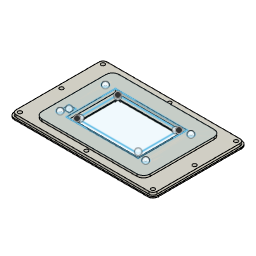
Display Mount - TFT35V20 (Autodesk Fusion 360 design; units mm, degrees)
Autodesk Fusion 360 part; units mm, degrees
note: some values were not read from the file. Set by a fixed rule: which sketch regions a step uses.
sketch "Sketch1" plane through (0, 0, 0) normal (0, 0, 1) x (1, 0, 0)
  circle A0 centre (-81.65, 51) radius 2.3
  circle A1 centre (81.65, 51) radius 2.3
  circle A2 centre (-81.65, -51) radius 2.3
  circle A3 centre (81.65, -51) radius 2.3
  line L0 (-81.65, 51) -> (81.65, 51) construction
  line L1 (81.65, 51) -> (81.65, -51) construction
  line L2 (81.65, -51) -> (-81.65, -51) construction
  line L3 (-81.65, -51) -> (-81.65, 51) construction
  circle A4 centre (-81.65, 0) radius 2.3
  circle A5 centre (0, 51) radius 2.3
  circle A6 centre (81.65, 0) radius 2.3
  circle A7 centre (0, -51) radius 2.3
  line L4 (0, 87.0412) -> (0, 82.962)
  line L5 (0, 82.962) -> (0, -82.962) construction
  line L6 (-123.3001, 0) -> (123.3001, 0) construction
  circle A8 centre (81.65, -51) radius 4.9
  circle A9 centre (-81.65, -51) radius 4.9
  circle A10 centre (-81.65, 51) radius 4.9
  circle A11 centre (81.65, 51) radius 4.9
  line L7 (-81.65, 55.9) -> (81.65, 55.9)
  line L8 (86.55, 51) -> (86.55, -51)
  line L9 (-81.65, -55.9) -> (-65.5347, -55.9)
  line L10 (-65.5347, -55.9) -> (81.65, -55.9)
  line L11 (-86.55, 51) -> (-86.55, -51)
  point P0 (0, 51)
  point P1 (81.65, 0)
  point P2 (0, -51)
  point P3 (-81.65, 0)
  dimension "d23" = 4.6
  dimension "d24" = 4.6
  dimension "d25" = 4.6
  dimension "d26" = 4.6
  dimension "d92" = 4.6
  dimension "d93" = 4.6
  dimension "d94" = 4.6
  dimension "d95" = 4.6
  dimension "d178" = 163.3
  dimension "d179" = 102
  dimension "d180" = 9.8
  dimension "d181" = 9.8
  dimension "d182" = 9.8
  dimension "d183" = 9.8
  constraint coincident A0.centre L0.start
  constraint coincident A3.centre L1.end
  constraint coincident A2.centre L2.end
  constraint midpoint L0 P0
  constraint midpoint L1 P1
  constraint midpoint L2 P2
  constraint midpoint L3 P3
  constraint coincident P3 A4.centre
  constraint coincident P0 A5.centre
  constraint coincident P1 A6.centre
  constraint coincident P2 A7.centre
  constraint midpoint origin L6
  constraint midpoint origin L5
  constraint symmetric A0.centre A1.centre L5
  constraint vertical A0.centre P3
  constraint symmetric A0.centre A2.centre L6
  constraint coincident P1 L6
  constraint parallel L0 L2
  constraint parallel L1 L3
  constraint coincident P0 L5
  constraint concentric A3 A8
  constraint concentric A2 A9
  constraint concentric A0 A10
  constraint concentric A1 A11
  constraint coincident A10 L7.start
  constraint coincident A11 L7.end
  constraint parallel L0 L7
  constraint tangent A11 L7
  constraint coincident A11 L8.start
  constraint coincident A8 L8.end
  constraint vertical L8
  constraint tangent A8 L8
  constraint coincident A9 L9.start
  constraint tangent A9 L9
  constraint perpendicular L5 L9
  constraint coincident A8 L10.end
  constraint tangent A8 L10
  constraint perpendicular L5 L10
  constraint coincident A10 L11.start
  constraint coincident A9 L11.end
  constraint tangent A9 L11
  constraint tangent A10 L11
  measures "d23" diameter of A0
  measures "d24" diameter of A1
  measures "d25" diameter of A2
  measures "d26" diameter of A3
  measures "d92" diameter of A4
  measures "d93" diameter of A7
  measures "d94" diameter of A6
  measures "d95" diameter of A5
  measures "d178" distance of A0.centre A1.centre
  measures "d179" distance of A0.centre A2.centre
  measures "d180" diameter of A8
  measures "d181" diameter of A9
  measures "d182" diameter of A10
  measures "d183" diameter of A11
extrude "Extrude1" add sketch "Sketch1" along normal blind 3
sketch "Sketch6" plane through (0, 0, 3) normal (0, 0, 1) x (-1, 0, 0)
  circle A0 centre (-81.65, 51) radius 2.3
  circle A1 centre (-81.65, -51) radius 2.3
  circle A2 centre (81.65, -51) radius 2.3
  circle A3 centre (81.65, 51) radius 2.3
  line L0 (0, -100) -> (0, 100) construction
  line L1 (148.8555, 0) -> (144.6445, 0)
  line L2 (144.6445, 0) -> (-144.6445, 0) construction
  line L3 (66.4, -47.3125) -> (-66.4, -47.3125)
  line L4 (-66.4, -47.3125) -> (-66.4, 47.3125)
  line L5 (-66.4, 47.3125) -> (66.4, 47.3125)
  line L6 (66.4, 47.3125) -> (66.4, -47.3125)
  circle A4 centre (0, 51) radius 2.3
  circle A5 centre (81.65, 0) radius 2.3
  circle A6 centre (0, -51) radius 2.3
  circle A7 centre (-81.65, 0) radius 2.3
  arc A8 (-81.65, 55.9) -> (-86.55, 51) centre (-81.65, 51) ccw
  arc A9 (-86.55, -51) -> (-81.65, -55.9) centre (-81.65, -51) ccw
  arc A10 (81.65, -55.9) -> (86.55, -51) centre (81.65, -51) ccw
  arc A11 (86.55, 51) -> (81.65, 55.9) centre (81.65, 51) ccw
  line L7 (-81.65, -55.9) -> (81.65, -55.9)
  line L8 (86.55, -51) -> (86.55, 51)
  line L9 (81.65, 55.9) -> (-81.65, 55.9)
  line L10 (-86.55, 51) -> (-86.55, -51)
  constraint vertical L0
  constraint horizontal L1
  constraint midpoint origin L2
  constraint midpoint origin L0
  constraint horizontal L3
  constraint vertical L4
  constraint horizontal L5
  constraint vertical L6
  constraint symmetric L0 L4 L6
  constraint symmetric L2 L3 L5
extrude "Extrude7" add sketch "Sketch6" along normal blind 2.6 contours L3 L4 L5 L6
fillet "Fillet2" radius 8 4 edges at (-66.4, -47.3125, 4.3) (66.4, -47.3125, 4.3) (66.4, 47.3125, 4.3) (-66.4, 47.3125, 4.3)
sketch "Sketch8" plane through (0, 0, 0) normal (0, 0, -1) x (1, 0, 0)
  circle A0 centre (81.65, 51) radius 2.3
  circle A1 centre (0, 51) radius 2.3
  circle A2 centre (-81.65, 0) radius 2.3
  circle A3 centre (-81.65, 51) radius 2.3
  circle A4 centre (81.65, -51) radius 2.3
  circle A5 centre (0, -51) radius 2.3
  circle A6 centre (-81.65, -51) radius 2.3
  circle A7 centre (81.65, 0) radius 2.3
  line L0 (81.65, 57.9) -> (-81.65, 57.9)
  line L1 (-88.55, 51) -> (-88.55, -51)
  line L2 (-81.65, -57.9) -> (81.65, -57.9)
  line L3 (88.55, -51) -> (88.55, 51)
  arc A8 (86.55, 51) -> (81.65, 55.9) centre (81.65, 51) ccw
  arc A9 (-81.65, 55.9) -> (-86.55, 51) centre (-81.65, 51) ccw
  arc A10 (-86.55, -51) -> (-81.65, -55.9) centre (-81.65, -51) ccw
  arc A11 (81.65, -55.9) -> (86.55, -51) centre (81.65, -51) ccw
  line L4 (86.55, -51) -> (86.55, 51)
  line L5 (81.65, 55.9) -> (-81.65, 55.9)
  line L6 (-86.55, 51) -> (-86.55, -51)
  line L7 (-81.65, -55.9) -> (81.65, -55.9)
  circle A12 centre (81.65, 51) radius 6.9
  circle A13 centre (-81.65, 51) radius 6.9
  circle A14 centre (-81.65, -51) radius 6.9
  circle A15 centre (81.65, -51) radius 6.9
  dimension "d184" = 2
  dimension "d185" = 2
  dimension "d186" = 2
  dimension "d187" = 2
  constraint concentric A0 A12
  constraint tangent L3 A12
  constraint tangent L0 A13
  constraint tangent L1 A13
  constraint coincident A3.centre A9.centre
  constraint tangent L1 A14
  constraint tangent L2 A14
  constraint coincident A6.centre A10.centre
  constraint tangent L2 A15
  constraint tangent L3 A15
  constraint coincident A4.centre A11.centre
  constraint coincident L0.end A13
  constraint coincident L0.start A12
  constraint coincident L2.end A15
  constraint coincident L2.start A14
  constraint coincident L1.start A13
  constraint coincident L1.end A14
  constraint coincident L3.start A15
  constraint coincident L3.end A12
  measures "d184" distance of L1 L6
  measures "d185" distance of L0 L5
  measures "d186" distance of L3 L4
  measures "d187" distance of L2 L7
extrude "Extrude15" add sketch "Sketch8" along normal blind 2.4
fillet "Fillet5" radius 1 8 edges at (88.55, 0, -2.4) (86.529, -55.879, -2.4) (0, -57.9, -2.4) (-86.529, -55.879, -2.4) (-88.55, 0, -2.4) (-86.529, 55.879, -2.4) (0, 57.9, -2.4) (86.529, 55.879, -2.4)
sketch "Sketch10" plane through (0, 0, 5.6) normal (0, 0, 1) x (-1, 0, 0)
  arc A0 (58.4, -47.3125) -> (66.4, -39.3125) centre (58.4, -39.3125) ccw
  line L0 (66.4, -39.3125) -> (66.4, 39.3125)
  arc A1 (66.4, 39.3125) -> (58.4, 47.3125) centre (58.4, 39.3125) ccw
  line L1 (58.4, 47.3125) -> (-58.4, 47.3125)
  arc A2 (-58.4, 47.3125) -> (-66.4, 39.3125) centre (-58.4, 39.3125) ccw
  line L2 (-66.4, 39.3125) -> (-66.4, -39.3125)
  arc A3 (-66.4, -39.3125) -> (-58.4, -47.3125) centre (-58.4, -39.3125) ccw
  line L3 (-58.4, -47.3125) -> (58.4, -47.3125)
  line L4 (35.5, -25) -> (-35.5, -25)
  line L5 (-37.5, -23) -> (-37.5, 23)
  line L6 (-35.5, 25) -> (35.5, 25)
  line L7 (37.5, 23) -> (37.5, -23)
  circle A4 centre (55.5, 27.75) radius 1.375
  circle A5 centre (55.5, 27.75) radius 3.5
  circle A6 centre (55.5, -27.75) radius 1.375
  circle A7 centre (55.5, -27.75) radius 3.5
  circle A8 centre (-49.5, -27.75) radius 1.375
  circle A9 centre (-49.5, -27.75) radius 3.5
  circle A10 centre (-49.5, 27.75) radius 1.375
  circle A11 centre (-49.5, 27.75) radius 3.5
  line L8 (45.5, -30) -> (-42.5, -30)
  line L9 (-42.5, -30) -> (-42.5, 30)
  line L10 (-42.5, 30) -> (45.5, 30)
  line L11 (56.5, 15.7496) -> (48.5, 15.7496)
  line L12 (48.5, 15.7496) -> (48.5, 23.7496)
  line L13 (48.5, 23.7496) -> (56.5, 23.7496)
  line L14 (56.5, 23.7496) -> (56.5, 15.7496)
  arc A12 (35.5, -25) -> (37.5, -23) centre (35.5, -23) ccw
  arc A13 (-37.5, -23) -> (-35.5, -25) centre (-35.5, -23) ccw
  arc A14 (-35.5, 25) -> (-37.5, 23) centre (-35.5, 23) ccw
  arc A15 (37.5, 23) -> (35.5, 25) centre (35.5, 23) ccw
  circle A16 centre (52.5, 19.75) radius 2.25
  line L15 (45.5, -30) -> (45.5, 30)
  point P0 (37.5, -25)
  point P1 (-37.5, -25)
  point P2 (37.5, 25)
  dimension "d31" = 75
  dimension "d32" = 50
  dimension "d33" = 105
  dimension "d34" = 55.5
  dimension "d38" = 2.75
  dimension "d39" = 7
  dimension "d40" = 2.75
  dimension "d41" = 7
  dimension "d42" = 2.75
  dimension "d43" = 7
  dimension "d44" = 2.75
  dimension "d45" = 7
  dimension "d76" = 8
  dimension "d77" = 8
  dimension "d78" = 2
  dimension "d80" = 4.5
  constraint horizontal L4
  constraint vertical L5
  constraint horizontal L6
  constraint vertical L7
  constraint concentric A4 A5
  constraint concentric A6 A7
  constraint concentric A8 A9
  constraint concentric A10 A11
  constraint horizontal L8
  constraint vertical L9
  constraint horizontal L10
  constraint horizontal L11
  constraint vertical L12
  constraint horizontal L13
  constraint vertical L14
  constraint coincident P0 L4
  constraint coincident P0 L7
  constraint tangent L4 A12
  constraint tangent L7 A12
  constraint coincident P1 L4
  constraint coincident P1 L5
  constraint tangent L4 A13
  constraint tangent L5 A13
  constraint equal A12 A13
  constraint tangent L5 A14
  constraint tangent L6 A14
  constraint equal A12 A14
  constraint coincident P2 L6
  constraint coincident P2 L7
  constraint tangent L6 A15
  constraint tangent L7 A15
  constraint equal A12 A15
  constraint parallel L0 L15
  measures "d31" distance of P0 P1
  measures "d32" distance of P0 P2
  measures "d33" distance of A6.centre A8.centre
  measures "d34" distance of A4.centre A6.centre
  measures "d38" diameter of A4
  measures "d39" diameter of A5
  measures "d40" diameter of A6
  measures "d41" diameter of A7
  measures "d42" diameter of A8
  measures "d43" diameter of A9
  measures "d44" diameter of A10
  measures "d45" diameter of A11
  measures "d76" distance of L11.start L11.end
  measures "d77" distance of L11.start L13.end
  measures "d78" radius of A12
  measures "d80" diameter of A16
extrude "Extrude34" cut sketch "Sketch10" against normal blind 4 contours L8 L9 L10 L15
extrude "Extrude31" cut sketch "Sketch10" against normal blind 8 draft -5 contours A16
extrude "Extrude18" cut sketch "Sketch10" against normal blind 10 contours L4 L5 L6 L7 A12 A13 A14 A15
extrude "Extrude23" cut sketch "Sketch10" against normal blind 5 contours A4
extrude "Extrude25" cut sketch "Sketch10" against normal blind 5 contours A6
extrude "Extrude27" cut sketch "Sketch10" against normal blind 5 contours A8
extrude "Extrude29" cut sketch "Sketch10" against normal blind 5 contours A10
fillet "Fillet7" radius 3 8 edges at (37.5, 0, -2.4) (36.9142, 24.4142, -2.4) (0, 25, -2.4) (-36.9142, 24.4142, -2.4) (-37.5, 0, -2.4) (-36.9142, -24.4142, -2.4) (0, -25, -2.4) (36.9142, -24.4142, -2.4)
extrude "Extrude32" cut sketch "Sketch10" against normal blind 6 contours L11 L12 L13 L14
extrude "Extrude33" cut sketch "Sketch10" against normal blind 8 contours A16
equation "d24 = d23"
equation "d25 = d23"
equation "d26 = d23"
equation "d92 = d23"
equation "d93 = d23"
equation "d94 = d23"
equation "d95 = d23"
equation "d178 = 173.2 mm - 9.9 mm"
equation "d180 = d181"
equation "d182 = d181"
equation "d183 = d181"
